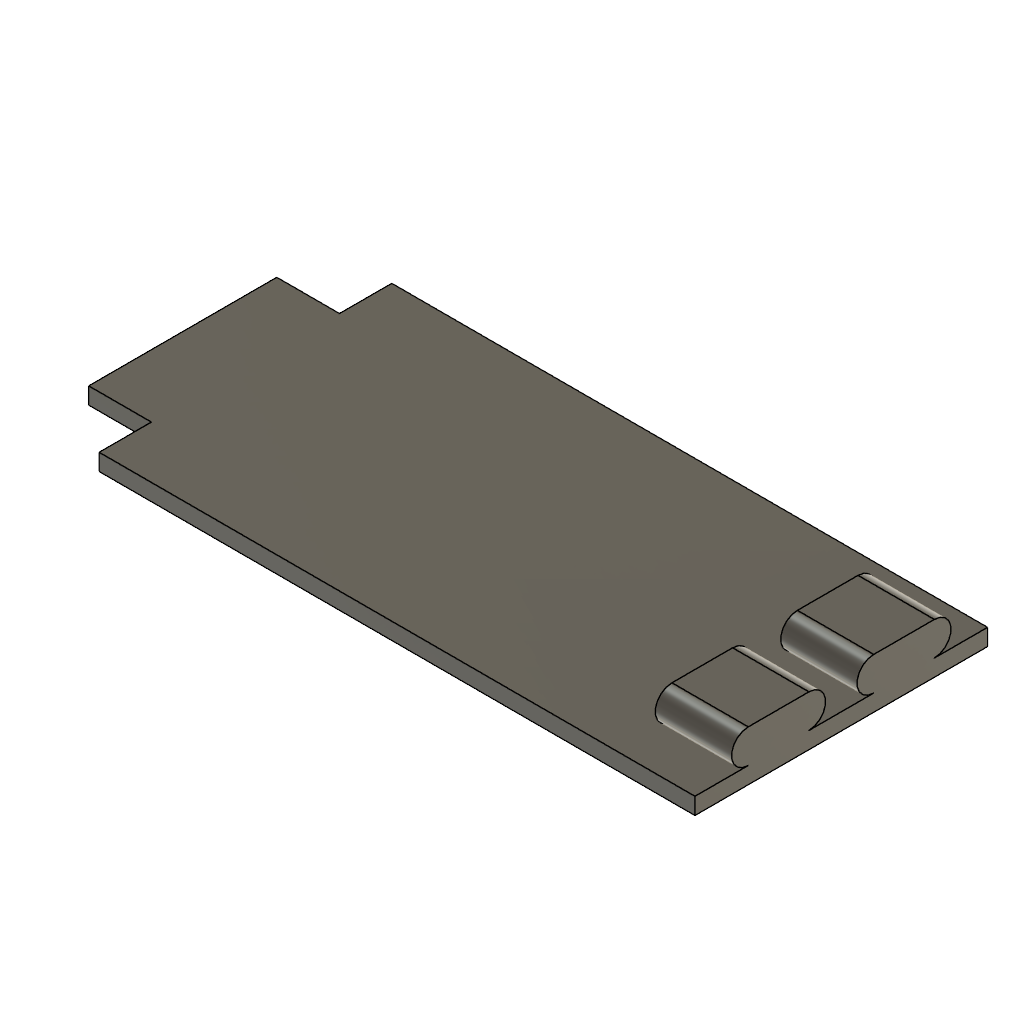
ZSB ESP32-Bridge (Autodesk Fusion 360 archive; units mm, degrees)
design "ESP32-S3"
Autodesk Fusion 360 part; units mm, degrees
sketch "Skizze1" plane through (0, 0, 0) normal (0, 0, 1) x (1, 0, 0)
  line L0 (0, 0) -> (-57, 0)
  line L1 (-57, 0) -> (-57, 28)
  line L2 (-57, 28) -> (0, 28)
  line L3 (0, 28) -> (0, 0)
  line L4 (-57, 23) -> (-63, 23)
  line L5 (-63, 23) -> (-63, 5)
  line L6 (-63, 5) -> (-57, 5)
  line L7 (-57, 5) -> (-57, 23)
  line L8 (0, 14) -> (-57, 14) construction
  dimension "d1" = 57
  dimension "d2" = 28
  dimension "d3" = 6
  dimension "d4" = 18
  constraint horizontal L0
  constraint vertical L1
  constraint horizontal L2
  constraint vertical L3
  constraint coincident L0.start L3.end
  constraint horizontal L4
  constraint vertical L5
  constraint horizontal L6
  constraint vertical L7
  constraint coincident L1 L4.start
  constraint midpoint L3 L8.start
  constraint coincident L1 L8.end
  constraint horizontal L8
  constraint symmetric L4 L6 L8
  measures "d1" distance of L1.end L2.end
  measures "d2" distance of L0.end L1.end
  measures "d3" distance of L4.start L4.end
  measures "d4" distance of L4.end L6
extrude "Extrusion1" add sketch "Skizze1" along normal blind 1.6
sketch "Skizze2" plane through (0, 0, 0) normal (1, 0, 0) x (0, 1, 0)
  line L0 (0, 0) -> (28, 0)
  line L1 (28, 0) -> (28, 1.6)
  line L2 (28, 1.6) -> (0, 1.6)
  line L3 (0, 1.6) -> (0, 0)
  line L4 (23, 1.6) -> (5, 1.6)
  line L5 (5, 1.6) -> (0, 1.6)
  line L6 (0, 1.6) -> (28, 1.6)
  line L7 (28, 1.6) -> (23, 1.6)
  line L8 (5.1, 4.8) -> (10.9, 4.8)
  line L9 (10.9, 1.6) -> (5.1, 1.6)
  line L10 (17.1, 4.8) -> (22.9, 4.8)
  line L11 (17.1, 1.6) -> (22.9, 1.6)
  arc A0 (5.1, 4.8) -> (5.1, 1.6) centre (5.1, 3.2) ccw
  arc A1 (10.9, 1.6) -> (10.9, 4.8) centre (10.9, 3.2) ccw
  arc A2 (17.1, 4.8) -> (17.1, 1.6) centre (17.1, 3.2) ccw
  arc A3 (22.9, 1.6) -> (22.9, 4.8) centre (22.9, 3.2) ccw
  line L12 (14, 1.6) -> (14, 0) construction
  dimension "d7" = 3.2
  dimension "d8" = 3.2
  dimension "d9" = 5.8
  dimension "d10" = 5.8
  dimension "d11" = 6.2
  constraint horizontal L10
  constraint horizontal L11
  constraint horizontal L8
  constraint horizontal L9
  constraint tangent L10 A3
  constraint tangent L10 A2
  constraint tangent L11 A2
  constraint tangent L11 A3
  constraint tangent L8 A1
  constraint tangent L8 A0
  constraint tangent L9 A0
  constraint tangent L9 A1
  constraint coincident L6 L9.start
  constraint coincident L2 L11.start
  constraint midpoint L6 L12.start
  constraint midpoint L0 L12.end
  constraint symmetric L9.start L11.start L12
  measures "d7" distance of L10 L11
  measures "d8" distance of L8 L9
  measures "d9" distance of A0.centre A1.centre
  measures "d10" distance of A2.centre A3.centre
  measures "d11" distance of A1.centre A2.centre
extrude "Extrusion2" add sketch "Skizze2" against normal blind 7.3 contours L2 L4 L6 L8 L9 A0 A1 | L2 L4 L6 L10 L11 A2 A3
sketch "Skizze3" plane through (0, 0, 0) normal (0, 0, -1) x (1, 0, 0)
  line L0 (-63, -23) -> (-57, -23)
  line L1 (-57, -23) -> (-57, -28)
  line L2 (-57, -28) -> (0, -28)
  line L3 (0, -28) -> (0, 0)
  line L4 (0, 0) -> (-57, 0)
  line L5 (-57, 0) -> (-57, -5)
  line L6 (-57, -5) -> (-63, -5)
  line L7 (-63, -5) -> (-63, -23)
  line L8 (0, -26.7) -> (-57, -26.7) construction
  line L9 (0, -1.3) -> (-57, -1.3) construction
  line L10 (-1.83, -26.7) -> (-1.83, -1.3) construction
  line L11 (-55.17, -26.7) -> (-55.17, -1.3) construction
  line L12 (-1.83, -26.7) -> (0, -26.7) construction
  line L13 (-57, -26.7) -> (-55.17, -26.7) construction
  line L14 (0, -14) -> (-63, -14) construction
  point P0 (-1.83, -1.3)
  point P1 (-55.17, -1.3)
  point P2 (-55.17, -26.7)
  point P3 (-1.83, -26.7)
  dimension "d14" = 53.34
  dimension "d16" = 25.4
  constraint coincident L3 L8.start
  constraint coincident L1 L8.end
  constraint coincident L3 L9.start
  constraint coincident L5 L9.end
  constraint horizontal L9
  constraint horizontal L8
  constraint coincident L9 P0
  constraint coincident L9 P1
  constraint coincident L8 P2
  constraint coincident L8 P3
  constraint coincident P3 L10.start
  constraint coincident P2 L11.start
  constraint vertical L10
  constraint vertical L11
  constraint coincident P0 L10.end
  constraint coincident P1 L11.end
  constraint equal L12 L13
  constraint midpoint L3 L14.start
  constraint midpoint L7 L14.end
  constraint symmetric P0 P3 L14
  measures "d14" distance of L10 L11
  measures "d16" distance of L8 L9
equation "d8 = d7"
equation "d9 = d10"
equation "d10 = 9 mm - 3.2 mm"
equation "d11 = 3 mm + 3.2 mm"
equation "d14 = ( 21 * 2.54 ) * 1 mm"
equation "d16 = ( 10 * 2.54 ) * 1 mm"

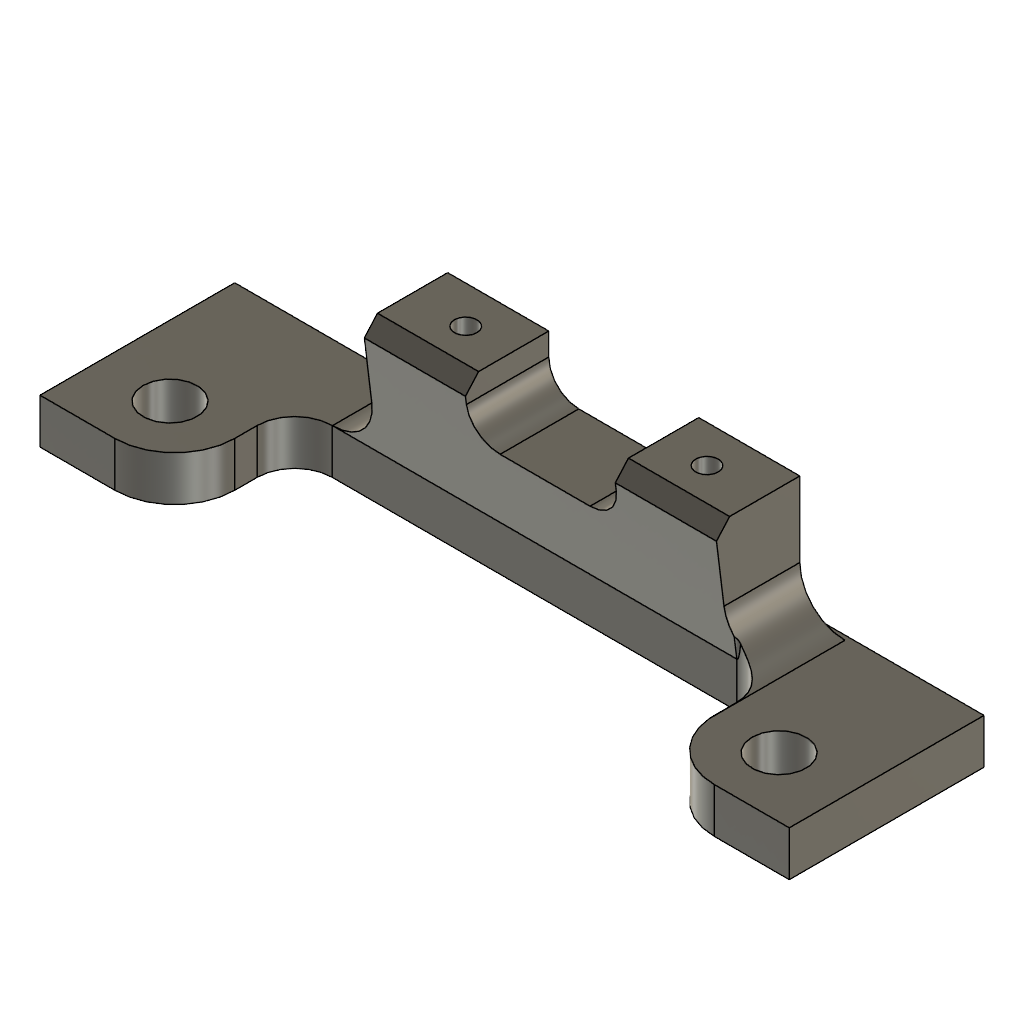
design "Traeger"
Autodesk Fusion 360 part; units mm, degrees
sketch "Skizze1" plane through (0, 0, 0) normal (0, 0, 1) x (1, 0, 0)
  line L0 (0, 0) -> (-50, 0)
  line L1 (-50, 0) -> (-50, 13)
  line L2 (-50, 13) -> (0, 13)
  line L3 (0, 13) -> (0, 0)
  circle A0 centre (-4.68, 4) radius 1.8
  circle A1 centre (-45.32, 4) radius 1.8
  line L4 (-50, 4) -> (0, 4) construction
  line L5 (-25, 13) -> (-25, 0) construction
  line L6 (-41, 0) -> (-41, 8)
  line L7 (-41, 8) -> (-9, 8)
  line L8 (-9, 8) -> (-9, 0)
  dimension "d1" = 50
  dimension "d2" = 13
  dimension "d3" = 3.6
  dimension "d4" = 40.64
  dimension "d5" = 9
  dimension "d11" = 5
  dimension "d12" = 9
  dimension "d13" = 9
  constraint horizontal L0
  constraint vertical L1
  constraint horizontal L2
  constraint vertical L3
  constraint coincident L0.start L3.end
  constraint coincident L1 L4.start
  constraint coincident L3 L4.end
  constraint perpendicular L3 L4
  constraint coincident A1.centre L4
  constraint coincident A0.centre L4
  constraint equal A0 A1
  constraint midpoint L2 L5.start
  constraint midpoint L0 L5.end
  constraint symmetric A0.centre A1.centre L5
  constraint coincident L0 L6.start
  constraint perpendicular L4 L6
  constraint perpendicular L6 L7
  constraint coincident L0 L8.end
  constraint perpendicular L0 L8
  measures "d1" distance of L0.start L0.end
  measures "d2" distance of L0.end L1.end
  measures "d3" diameter of A1
  measures "d4" distance of A0.centre A1.centre
  measures "d5" distance of L2 L4
  measures "d11" distance of L2 L7
  measures "d12" distance of L1 L6
  measures "d13" distance of L3 L8
extrude "Extrusion1" add sketch "Skizze1" along normal blind 3 contours L0 L1 L2 L3 L6 L7 L8
sketch "Skizze2" plane through (0, 0, 3) normal (0, 0, 1) x (-1, 0, 0)
  circle A0 centre (4.68, -4) radius 1.8
  circle A1 centre (45.32, -4) radius 1.8
  line L0 (41, 0) -> (41, -8)
  line L1 (41, -8) -> (9, -8)
  line L2 (9, 0) -> (0, 0)
  line L3 (0, 0) -> (0, -13)
  line L4 (0, -13) -> (50, -13)
  line L5 (50, -13) -> (50, 0)
  line L6 (50, 0) -> (41, 0)
  line L7 (34.48, -0.19) -> (12.98, -0.19) construction
  line L8 (12.98, -0.19) -> (12.98, -12.69) construction
  line L9 (12.98, -12.69) -> (34.48, -12.69) construction
  line L10 (34.48, -12.69) -> (34.48, -0.19) construction
  circle A2 centre (31.78, -10.19) radius 0.75
  circle A3 centre (15.68, -10.19) radius 0.75
  line L11 (34.48, -10.19) -> (12.98, -10.19) construction
  line L12 (31.78, -12.69) -> (31.78, -0.19) construction
  line L13 (15.68, -12.69) -> (15.68, -0.19) construction
  line L14 (34.48, -1.46) -> (12.98, -1.46) construction
  line L15 (23.73, -12.69) -> (23.73, -0.19) construction
  line L16 (35.48, -8) -> (35.48, -13)
  line L17 (11.98, -8) -> (11.98, -13)
  line L18 (11.98, -12.69) -> (35.48, -12.69)
  point P0 (30.08, -1.46)
  point P1 (17.38, -1.46)
  dimension "d20" = 1.5
  dimension "d21" = 1.5
  dimension "d22" = 21.5
  dimension "d23" = 12.5
  dimension "d25" = 2.5
  dimension "d27" = 1.27
  dimension "d28" = 12.7
  dimension "d29" = 15.24
  dimension "d30" = 12.7
  dimension "d31" = 2.54
  dimension "d32" = 1
  dimension "d33" = 1
  dimension "d51" = 16.1
  constraint horizontal L7
  constraint vertical L8
  constraint horizontal L9
  constraint vertical L10
  constraint coincident L10 L11.start
  constraint coincident L8 L11.end
  constraint perpendicular L8 L11
  constraint coincident L9 L12.start
  constraint coincident L7 L12.end
  constraint perpendicular L7 L12
  constraint coincident L9 L13.start
  constraint coincident L7 L13.end
  constraint perpendicular L7 L13
  constraint coincident A2.centre L11
  constraint coincident A2.centre L12
  constraint coincident A3.centre L13
  constraint coincident A3.centre L11
  constraint coincident L10 L14.start
  constraint coincident L8 L14.end
  constraint perpendicular L8 L14
  constraint coincident L14 P0
  constraint coincident L14 P1
  constraint midpoint L9 L15.start
  constraint midpoint L7 L15.end
  constraint symmetric P0 P1 L15
  constraint coincident L1 L16.start
  constraint coincident L4 L16.end
  constraint coincident L1 L17.start
  constraint coincident L4 L17.end
  constraint vertical L17
  constraint vertical L16
  constraint coincident L17 L18.start
  constraint coincident L16 L18.end
  constraint perpendicular L16 L18
  constraint coincident L8.end L18
  constraint symmetric A2.centre A3.centre L15
  measures "d20" diameter of A2
  measures "d21" diameter of A3
  measures "d22" distance of L7.start L7.end
  measures "d23" distance of L7.start L9.end
  measures "d25" distance of L9 L11
  measures "d27" distance of L7 L14
  measures "d28" distance of P0 P1
  measures "d29" horizontal distance of A1.centre P0
  measures "d30" horizontal distance of A0.centre P1
  measures "d31" vertical distance of A1.centre P0
  measures "d32" distance of L8 L17
  measures "d33" distance of L10 L16
  measures "d51" distance of A2.centre A3.centre
extrude "Extrusion2" add sketch "Skizze2" along normal blind 8 contours L1 L16 L17 L18
sketch "Skizze3" plane through (0, 12.69, 0) normal (0, 1, 0) x (-1, 0, 0)
  line L0 (11.98, 3) -> (35.48, 3)
  line L1 (35.48, 3) -> (35.48, 11)
  line L2 (35.48, 11) -> (11.98, 11)
  line L3 (11.98, 11) -> (11.98, 3)
  line L4 (23.73, 11) -> (23.73, 2.7366) construction
  line L5 (18.73, 7.5) -> (28.73, 7.5)
  line L6 (28.73, 7.5) -> (28.73, 11)
  line L7 (18.73, 7.5) -> (18.73, 11)
  line L8 (18.73, 11) -> (28.73, 11)
  dimension "d37" = 3.5
  dimension "d38" = 10
  constraint midpoint L2 L4.start
  constraint perpendicular L0 L4
  constraint perpendicular L4 L5
  constraint coincident L2 L6.end
  constraint coincident L2 L7.end
  constraint symmetric L4 L6.end L7.end
  constraint symmetric L4 L5.start L5.end
  constraint vertical L7
  measures "d37" distance of L5 L8
  measures "d38" distance of L5.start L5.end
extrude "Extrusion3" cut sketch "Skizze3" against normal up to surface (4.69 mm away) contours L2 L5 L6 L7 L8
fillet "Abrundung1" radius 3 1 edges at (-11.98, 10.345, 3)
fillet "Abrundung2" radius 3 1 edges at (-35.48, 10.345, 3)
fillet "Abrundung3" radius 2 2 edges at (-18.73, 10.345, 7.5) (-28.73, 10.345, 7.5)
fillet "Abrundung4" radius 4 2 edges at (-9, 0, 1.5) (-41, 0, 1.5)
fillet "Abrundung5" radius 2.5 2 edges at (-9, 8, 1.5) (-41, 8, 1.5)
extrude "Extrusion4" add 1 faces at (-25.5767, 8, 2.5) along direction (0, -1, 0) blind 1
sketch "Skizze4" plane through (-38.5, 0, 0) normal (-1, 0, 0) x (0, -1, 0)
  line L0 (-8, 3) -> (-8, 0)
  line L1 (-8, 0) -> (-7, 0)
  line L2 (-7, 0) -> (-7, 3)
  line L3 (-7, 3) -> (-8, 3)
  line L4 (-8, 3) -> (-7, 3)
  line L5 (-7, 11) -> (-12.69, 11)
  line L6 (-12.69, 11) -> (-7, 11)
  line L7 (-10.94, 11) -> (-9.44, 11)
  line L8 (-7, 3) -> (-7, 11)
  line L9 (-8, 3) -> (-7, 11)
  constraint coincident L0.start L3.end
  constraint coincident L2.end L3.start
  constraint coincident L5.start L6.end
extrude "Extrusion5" cut sketch "Skizze4" against normal up to surface (27 mm away)
fillet "Abrundung6" radius 0.3 1 edges at (-11.5, 8, 3.6861)
chamfer "Fase1" distance 1 angle 45 2 edges at (-32.105, 7, 11) (-15.355, 7, 11) tangent chain off
equation "d4 = ( 16 * 2.54 ) * 1 mm"
equation "d13 = d12"
equation "d25 = 1 mm + 1.5 mm"
equation "d27 = ( 2.54 / 2 ) * 1 mm"
equation "d28 = ( 2.54 * 5 ) * 1 mm"
equation "d29 = ( 6 * 2.54 ) * 1 mm"
equation "d34 = 11 mm - 3 mm"

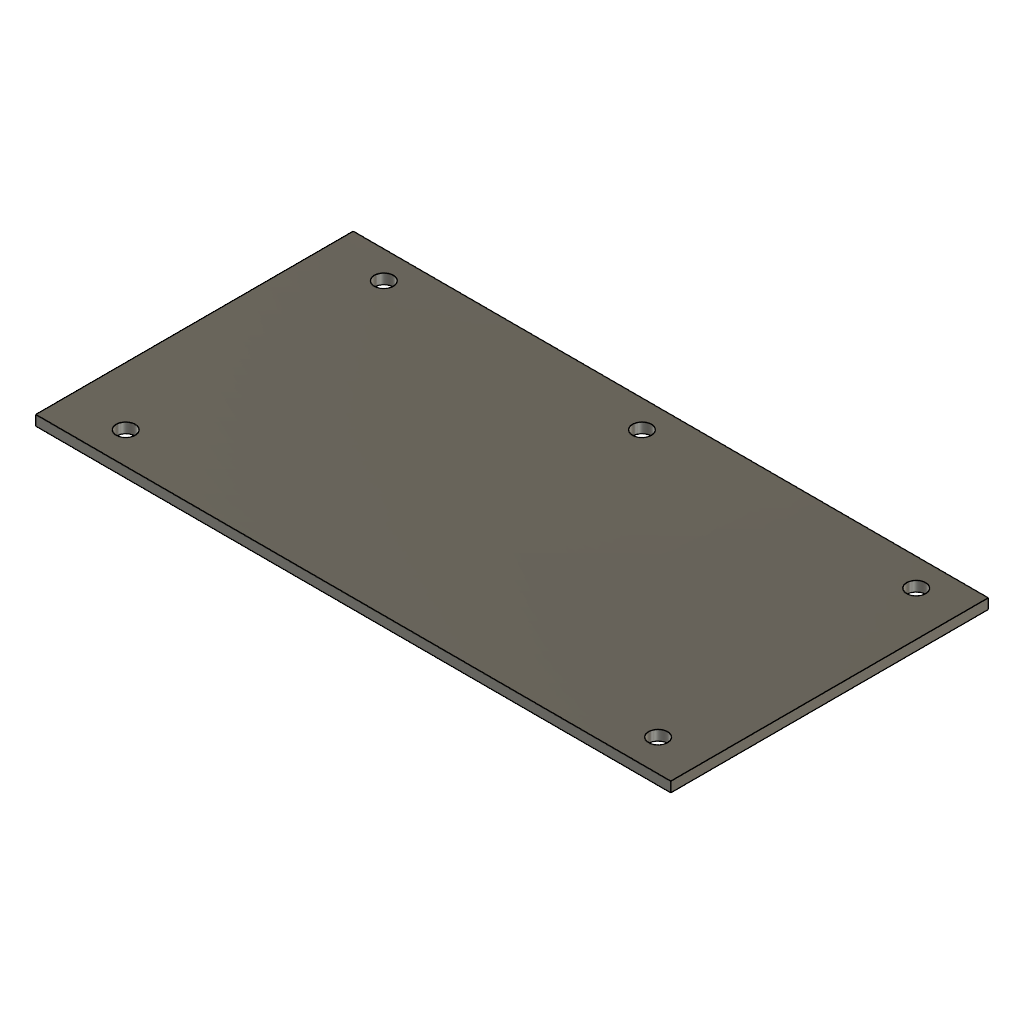
design "Platine"
Autodesk Fusion 360 part; units mm, degrees
sketch "Skizze1" plane through (0, 0, 0) normal (0, 0, 1) x (1, 0, 0)
  line L0 (-100, 50) -> (0, 50)
  line L1 (0, 50) -> (0, 0)
  line L2 (0, 0) -> (-100, 0)
  line L3 (-100, 0) -> (-100, 50)
  line L4 (-100, 45.64) -> (0, 45.64) construction
  line L5 (-100, 5) -> (0, 5) construction
  line L6 (-7, 50) -> (-7, 0) construction
  line L7 (-90.82, 50) -> (-90.82, 0) construction
  line L8 (-50.18, 50) -> (-50.18, 0) construction
  circle A0 centre (-90.82, 5) radius 1.5
  circle A1 centre (-90.82, 45.64) radius 1.5
  circle A2 centre (-7, 45.64) radius 1.5
  circle A3 centre (-7, 5) radius 1.5
  circle A4 centre (-50.18, 45.64) radius 1.5
  line L9 (-12.08, 50) -> (-12.08, 0) construction
  line L10 (-88.28, 50) -> (-88.28, 0) construction
  line L11 (-12.08, 20.24) -> (-88.28, 20.24) construction
  line L12 (-12.08, 32.94) -> (-88.28, 32.94) construction
  line L13 (-90.82, 12.62) -> (-7, 12.62) construction
  line L14 (-90.82, 38.02) -> (-7, 38.02) construction
  line L15 (-60.34, 38.02) -> (-60.34, 12.62) construction
  line L16 (-70.5, 45.64) -> (-70.5, 5) construction
  line L17 (-83.2, 45.64) -> (-83.2, 5) construction
  line L18 (-70.5, 35.48) -> (-83.2, 35.48) construction
  line L19 (-70.5, 15.16) -> (-83.2, 15.16) construction
  point P0 (-12.08, 20.24)
  point P1 (-12.08, 32.94)
  point P2 (-88.28, 32.94)
  point P3 (-88.28, 20.24)
  point P4 (-7, 38.02)
  point P5 (-7, 12.62)
  point P6 (-60.34, 38.02)
  point P7 (-60.34, 12.62)
  point P8 (-70.5, 35.48)
  point P9 (-70.5, 15.16)
  point P10 (-83.2, 15.16)
  point P11 (-83.2, 35.48)
  dimension "d1" = 100
  dimension "d2" = 50
  dimension "d3" = 5
  dimension "d4" = 7
  dimension "d5" = 83.82
  dimension "d6" = 40.64
  dimension "d7" = 3
  dimension "d9" = 5.08
  dimension "d10" = 2.54
  dimension "d11" = 12.7
  dimension "d14" = 25.4
  dimension "d15" = 5.08
  dimension "d16" = 12.7
  dimension "d17" = 53.34
  dimension "d19" = 10.16
  dimension "d20" = 12.7
  dimension "d21" = 2.54
  dimension "d22" = 2.54
  dimension "d29" = 40.64
  constraint horizontal L0
  constraint vertical L1
  constraint horizontal L2
  constraint vertical L3
  constraint coincident L1.end L2.start
  constraint coincident L3 L4.start
  constraint perpendicular L3 L4
  constraint coincident L3 L5.start
  constraint coincident L1 L5.end
  constraint perpendicular L1 L5
  constraint coincident L0 L6.start
  constraint coincident L2 L6.end
  constraint perpendicular L2 L6
  constraint coincident L0 L7.start
  constraint coincident L2 L7.end
  constraint perpendicular L2 L7
  constraint coincident L0 L8.start
  constraint coincident L2 L8.end
  constraint coincident L7 A0.centre
  constraint coincident L5 A0.centre
  constraint coincident L7 A1.centre
  constraint coincident L4 A1.centre
  constraint coincident L6 A2.centre
  constraint coincident L4 A2.centre
  constraint coincident L6 A3.centre
  constraint coincident L5 A3.centre
  constraint equal A2 A3
  constraint equal A1 A2
  constraint equal A0 A1
  constraint vertical L8
  constraint coincident L8 A4.centre
  constraint coincident L4 A4.centre
  constraint equal A2 A4
  constraint coincident L0 L9.start
  constraint coincident L2 L9.end
  constraint perpendicular L2 L9
  constraint coincident L0 L10.start
  constraint coincident L2 L10.end
  constraint perpendicular L2 L10
  constraint coincident L9 P0
  constraint coincident L9 P1
  constraint coincident P0 L11.start
  constraint coincident L10 P3
  constraint perpendicular L10 L11
  constraint coincident P1 L12.start
  constraint coincident L10 P2
  constraint perpendicular L10 L12
  constraint coincident P2 L12.end
  constraint coincident P3 L11.end
  constraint coincident L7 L13.start
  constraint coincident L6 P5
  constraint perpendicular L6 L13
  constraint coincident L7 L14.start
  constraint perpendicular L9 L14
  constraint coincident L6 P4
  constraint coincident P4 L14.end
  constraint coincident P5 L13.end
  constraint coincident L14 P6
  constraint coincident P6 L15.start
  constraint coincident L13 P7
  constraint perpendicular L13 L15
  constraint coincident P7 L15.end
  constraint coincident L4 L16.start
  constraint coincident L5 L16.end
  constraint perpendicular L5 L16
  constraint coincident L4 L17.start
  constraint coincident L5 L17.end
  constraint perpendicular L5 L17
  constraint coincident L16 P8
  constraint coincident L17 P11
  constraint perpendicular L17 L18
  constraint coincident L16 P9
  constraint coincident L17 P10
  constraint perpendicular L17 L19
  constraint coincident P8 L18.start
  constraint coincident P9 L19.start
  constraint coincident P10 L19.end
  constraint coincident P11 L18.end
  measures "d1" distance of L1.end L2.end
  measures "d2" distance of L0.end L1.end
  measures "d3" distance of L2 L5
  measures "d4" distance of L1 L6
  measures "d5" distance of L6 L7
  measures "d6" distance of L4 L5
  measures "d7" diameter of A3
  measures "d9" distance of L6 L9
  measures "d10" distance of L7 L10
  measures "d11" distance of P0 P1
  measures "d14" distance of L13 L14
  measures "d15" distance of L12 L14
  measures "d16" distance of L4 L12
  measures "d17" distance of P4 P6
  measures "d19" distance of P6 L16
  measures "d20" distance of L16 L17
  measures "d21" distance of L14 L18
  measures "d22" distance of L13 L19
  measures "d29" distance of A1.centre A4.centre
extrude "Extrusion1" add sketch "Skizze1" along normal blind 1.6
ref_plane "Arbeitsebene1" through (-50, 25, 12.6) normal (0, 0, 1) x (1, 0, 0)
sketch "Skizze2" plane through (0, 0, 12.6) normal (0, 0, 1) x (1, 0, 0)
  point P0 (-7, 38.02)
  point P1 (-7, 12.62)
  point P2 (-60.34, 38.02)
  point P3 (-60.34, 12.62)
  point P4 (-88.28, 32.94)
  point P5 (-88.28, 20.24)
ref_plane "Arbeitsebene2" through (-50, 25, -11) normal (0, 0, 1) x (1, 0, 0)
sketch "Skizze3" plane through (0, 0, -11) normal (0, 0, 1) x (1, 0, 0)
  point P0 (-83.2, 15.16)
  point P1 (-70.5, 15.16)
  point P2 (-70.5, 35.48)
  point P3 (-83.2, 35.48)
  point P4 (-12.08, 20.24)
  point P5 (-12.08, 32.94)
equation "d5 = 33 * 2.54 mm"
equation "d9 = ( 2 * 2.54 ) * 1 mm"
equation "d11 = ( 5 * 2.54 ) * 1 mm"
equation "d14 = ( 10 * 2.54 ) * 1 mm"
equation "d15 = 2 * 2.54 mm"
equation "d16 = ( 5 * 2.54 ) * 1 mm"
equation "d17 = ( 21 * 2.54 ) * 1 mm"
equation "d19 = ( 4 * 2.54 ) * 1 mm"
equation "d20 = ( 5 * 2.54 ) * 1 mm"
equation "d29 = ( 16 * 2.54 ) * 1 mm"

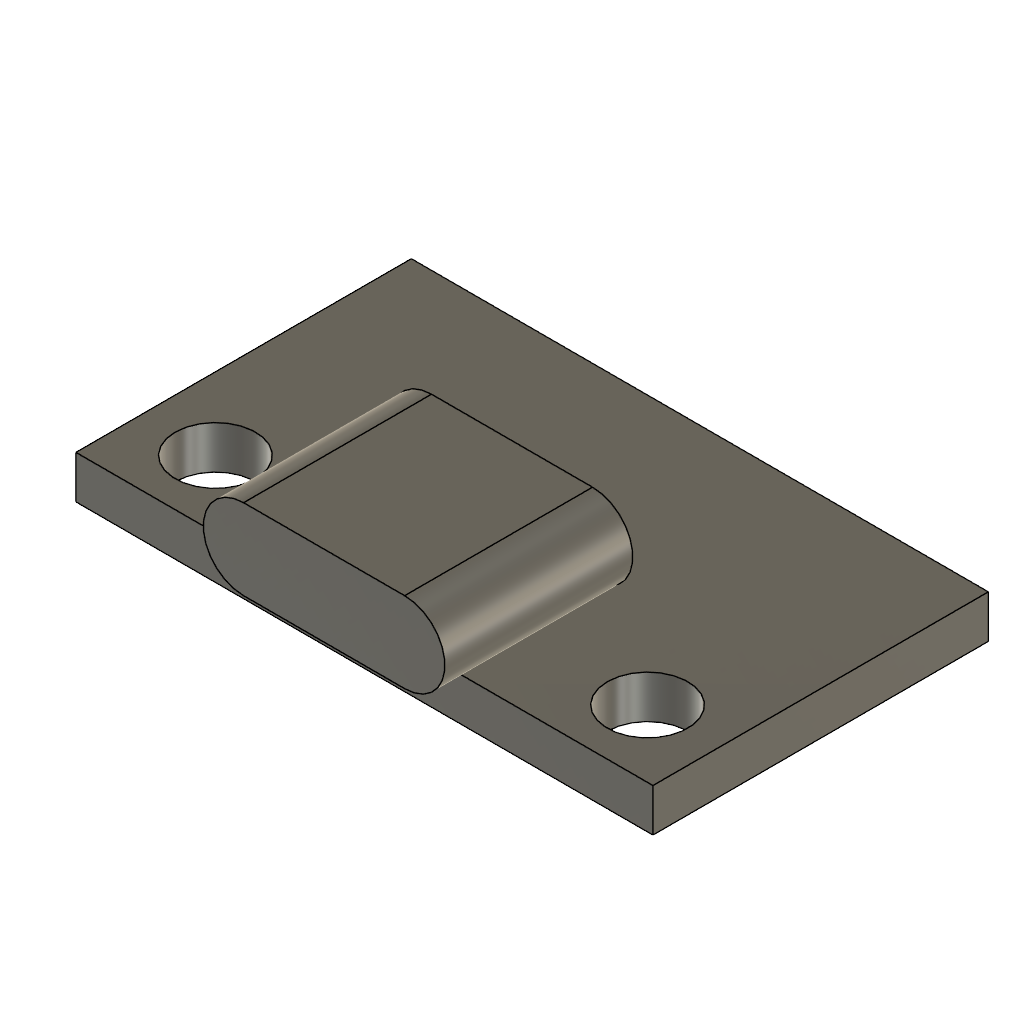
design "USB-Breakout"
Autodesk Fusion 360 part; units mm, degrees
sketch "Skizze1" plane through (0, 0, 0) normal (0, 0, 1) x (1, 0, 0)
  line L0 (0, 0) -> (-21.5, 0)
  line L1 (-21.5, 0) -> (-21.5, 12.5)
  line L2 (-21.5, 12.5) -> (0, 12.5)
  line L3 (0, 12.5) -> (0, 0)
  circle A0 centre (-18.8, 2.5) radius 1.5
  circle A1 centre (-2.7, 2.5) radius 1.5
  line L4 (-21.5, 11.23) -> (0, 11.23) construction
  line L5 (-10.75, 12.5) -> (-10.75, 0) construction
  point P0 (-10.75, 11.23)
  point P1 (-17.1, 11.23)
  point P2 (-4.4, 11.23)
  dimension "d1" = 21.5
  dimension "d2" = 12.5
  dimension "d3" = 3
  dimension "d4" = 2.7
  dimension "d5" = 2.7
  dimension "d6" = 2.5
  dimension "d7" = 2.5
  dimension "d8" = 1.27
  dimension "d19" = 12.7
  constraint horizontal L0
  constraint vertical L1
  constraint horizontal L2
  constraint vertical L3
  constraint coincident L0.start L3.end
  constraint equal A0 A1
  constraint coincident L1 L4.start
  constraint coincident L3 L4.end
  constraint perpendicular L3 L4
  constraint midpoint L2 L5.start
  constraint midpoint L0 L5.end
  constraint midpoint L4 P0
  constraint coincident L4 P1
  constraint coincident L4 P2
  constraint symmetric L5 P1 P2
  measures "d1" distance of L1.end L2.end
  measures "d2" distance of L0.end L1.end
  measures "d3" diameter of A0
  measures "d4" distance of L1 A0.centre
  measures "d5" distance of L3 A1.centre
  measures "d6" distance of L0 A0.centre
  measures "d7" distance of L0 A1.centre
  measures "d8" distance of L2 L4
  measures "d19" distance of P1 P2
extrude "Extrusion1" add sketch "Skizze1" along normal blind 1.6
sketch "Skizze2" plane through (0, 0, 0) normal (0, -1, 0) x (1, 0, 0)
  line L0 (-21.5, 0) -> (0, 0)
  line L1 (0, 0) -> (0, 1.6)
  line L2 (0, 1.6) -> (-21.5, 1.6)
  line L3 (-21.5, 1.6) -> (-21.5, 0)
  line L4 (-10.75, 0) -> (-10.75, 13.6465) construction
  line L5 (-13.75, 4.6) -> (-7.75, 4.6)
  line L6 (-7.75, 1.6) -> (-13.75, 1.6)
  arc A0 (-13.75, 4.6) -> (-13.75, 1.6) centre (-13.75, 3.1) ccw
  arc A1 (-7.75, 1.6) -> (-7.75, 4.6) centre (-7.75, 3.1) ccw
  point P0 (-10.75, 1.6)
  dimension "d11" = 1.5
  dimension "d12" = 6
  constraint midpoint L0 L4.start
  constraint perpendicular L2 L4
  constraint tangent L5 A1
  constraint tangent L6 A0
  constraint tangent L5 A0
  constraint tangent L6 A1
  constraint equal A0 A1
  constraint symmetric L4 L5.start L5.end
  constraint midpoint L2 P0
  constraint coincident L6 P0
  measures "d11" radius of A0
  measures "d12" distance of A0.centre A1.centre
extrude "Extrusion2" add sketch "Skizze2" along normal blind 1.5 and the other way blind 5.5 contours L2 L5 L6 A0 A1
sketch "Skizze3" plane through (0, 0, 1.6) normal (0, 0, 1) x (-1, 0, 0)
  line L0 (7.75, -5.5) -> (7.75, 0)
  line L1 (7.75, 0) -> (0, 0)
  line L2 (0, 0) -> (0, -12.5)
  line L3 (0, -12.5) -> (21.5, -12.5)
  line L4 (21.5, -12.5) -> (21.5, 0)
  line L5 (21.5, 0) -> (13.75, 0)
  line L6 (13.75, 0) -> (13.75, -5.5)
  line L7 (13.75, -5.5) -> (7.75, -5.5)
  circle A0 centre (2.7, -2.5) radius 1.5
  circle A1 centre (18.8, -2.5) radius 1.5
  point P0 (10.75, -11.23)
  point P1 (10.75, -11.23)
  point P2 (4.4, -11.23)
  point P3 (17.1, -11.23)
  constraint coincident P1 P0
ref_plane "Arbeitsebene1" through (0, 0, 5.1) normal (0, 0, 1) x (1, 0, 0)
sketch "Skizze4" plane through (0, 0, 5.1) normal (0, 0, 1) x (1, 0, 0)
  point P0 (-10.75, 11.23)
  point P1 (-10.75, 11.23)
  constraint coincident P0 P1
equation "d4 = 1.2 mm + 1.5 mm"
equation "d5 = d4"
equation "d7 = d6"
equation "d8 = ( 2.54 / 2 ) * 1 mm"
equation "d12 = 9 mm - 3 mm"
equation "d15 = 7 mm - 1.5 mm"
equation "d17 = 1.6 mm + 3.5 mm"
equation "d19 = ( 5 * 2.54 ) * 1 mm"
